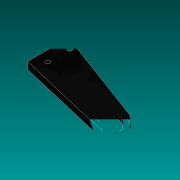
# Autodesk Inventor part: 胴体_サブフレーム_1_6
Saved by Autodesk Inventor 2016 (Build 200138000, 138)
## iProperties
Created: 2016-05-14
Part Number: 胴体_サブフレーム_1_6
Material: アセタール樹脂、黒
Document SubType Name: Modeling
Designer: hiroaki
Density: 1.425 g/cm^3
Appearance: 滑らか - 黒
Mass: 7.82787 g
Surface Area: 53.8383 cm^2
Volume: 5.49324 cm^3
Author: hiroaki
Autodesk Inventor part; units mm, degrees
ref_plane "YZ Plane" through (0, 0, 0) normal (1, 0, 0) x (0, 1, 0)
ref_plane "XZ Plane" through (0, 0, 0) normal (0, 1, 0) x (-1, 0, 0)
ref_plane "XY Plane" through (0, 0, 0) normal (0, 0, 1) x (1, 0, 0)
sketch "スケッチ1" plane through (0, 0, 0) normal (0, 0, 1) x (1, 0, 0)
  line L0 (-10.3125, 15) -> (-10.3125, -15)
  line L1 (-10.3125, -15) -> (0, -9.5)
  line L2 (0, -9.5) -> (0, 9.5)
  line L3 (0, 9.5) -> (-10.3125, 15)
  circle A0 centre (-2.5, 8) radius 1.55
  circle A1 centre (-2.5, -8) radius 1.55
  circle A2 centre (-2.5, 8) radius 2.5 construction
  circle A3 centre (-2.5, -8) radius 2.5 construction
  line L4 (-2.5, 8) -> (-2.5, -8) construction
  line L5 (-10.3125, 15) -> (59.873, -11.1505)
  line L6 (-10.3125, -15) -> (54.0766, -30.2519)
  arc A4 (54.0766, -30.2519) -> (59.873, -11.1505) centre (56.3816, -20.5212) ccw
  line L7 (56.3816, -20.5212) -> (0, 0) construction
  point P0 (-2.5, 0)
  dimension "d5" = 19
  dimension "d8" = 30
  dimension "d10" = 5
  dimension "d20" = 16
  dimension "d33" = 3.1
  dimension "d35" = 10
  dimension "d41" = 70
  dimension "d43" = 60
  constraints: 16 end point, 6 tangent, 5 centre point, 4 coincident, 2 equal radius, 2 midpoint, 2 point on circle, 2 vertical, 1 horizontal alignment, 1 parallel
  measures "d5" distance of L1.end L2.end
  measures "d8" distance of L0.start L0.end
  measures "d10" diameter of A2
  measures "d20" distance of L4.start L4.end
  measures "d33" diameter of A0
  measures "d35" radius of A4
  measures "d41" angle of L2 L7
  measures "d43" distance of L7.start L7.end
extrude "押し出し1" add sketch "スケッチ1" along normal blind 5
sketch "スケッチ4" plane through (0, 0, 0) normal (0, 0, -1) x (-1, 0, 0)
  circle A0 centre (2.5, 8) radius 1.55 projected
  line L0 (-59.873, -11.1505) -> (10.3125, 15) projected
  arc A1 (-59.873, -11.1505) -> (-54.0766, -30.2519) centre (-56.3816, -20.5212) ccw projected
  line L1 (10.3125, -15) -> (-54.0766, -30.2519) projected
  line L2 (-2.5, -13.9242) -> (-54.9986, -26.3597)
  arc A2 (-58.4764, -14.8988) -> (-54.9986, -26.3597) centre (-56.3816, -20.5212) ccw
  line L3 (-58.4764, -14.8988) -> (-2.5, 5.9575)
  line L4 (-2.5, -13.9242) -> (-2.5, 5.9575)
  point P0 (0, 0)
  dimension "d81" = 4
  dimension "d82" = 5
  constraints: 6 end point, 2 point on circle, 1 centre point, 1 vertical, 2 other
  measures "d81" distance between parallel lines of L0 L3
  measures "d82" distance from line of A0.centre L4
extrude "押し出し4" cut sketch "スケッチ4" against normal blind 4 contours L2 A2 L3 L4
fillet "フィレット4" radius 2 2 edges at (2.5, 5.9575, 2) (2.5, -13.9242, 2)
equation "\"d5\" = d187"
equation "\"d8\" = d98"
equation "\"d10\" = d185"
equation "\"d20\" = d186"
equation "\"d185\" = 5"
equation "\"d187\" = 19"
equation "\"d98\" = 30"
equation "\"d186\" = 16"
